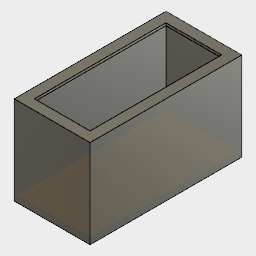
Doorbell_Casing_04 (Autodesk Fusion 360 design; units mm, degrees)
Autodesk Fusion 360 part; units mm, degrees
box "BoxPrimitive1" add length 60 width 30 height 35 placed x (0, 0, 1) y (1, 0, 0) z (0, 1, 0) at (0, 0, 0)
sketch "Sketch2" plane through (0, 35, 0) normal (0, 1, 0) x (-1, 0, 0)
  line L0 (0, 60) -> (-30, 60)
  line L1 (-30, 60) -> (-30, 0)
  line L2 (-30, 0) -> (0, 0)
  line L3 (0, 0) -> (0, 60)
  line L4 (-1, 0.9321) -> (-29, 0.9321)
  line L5 (-29, 0.9321) -> (-29, 58.9321)
  line L6 (-29, 58.9321) -> (-1, 58.9321)
  line L7 (-1, 58.9321) -> (-1, 0.9321)
  line L8 (-1, 0.9321) -> (-29, 58.9321) construction
  line L9 (-29, 0.9321) -> (-1, 58.9321) construction
  line L10 (-1, 58.9321) -> (-29, 58.9321)
  line L11 (-29, 58.9321) -> (-29, 0.9321)
  line L12 (-29, 0.9321) -> (-1, 0.9321)
  line L13 (-1, 0.9321) -> (-1, 58.9321)
  line L14 (30, 60) -> (0, 60)
  line L15 (0, 60) -> (0, 0)
  line L16 (0, 0) -> (30, 0)
  line L17 (30, 0) -> (30, 60)
  circle A0 centre (-15, 29.9346) radius 5
  line L18 (-1, 58.9321) -> (-29, 58.9321)
  line L19 (-29, 58.9321) -> (-29, 0.9321)
  line L20 (-29, 0.9321) -> (-1, 0.9321)
  line L21 (-1, 0.9321) -> (-1, 58.9321)
  circle A1 centre (15, 30) radius 4.5
  line L22 (30, 60) -> (0, 60)
  line L23 (0, 60) -> (0, 0)
  line L24 (0, 0) -> (30, 0)
  line L25 (30, 0) -> (30, 60)
  circle A2 centre (15, 40.0509) radius 2.5
  circle A3 centre (15, 30) radius 4.5
  line L26 (30, 60) -> (0, 60)
  line L27 (0, 60) -> (0, 0)
  line L28 (0, 0) -> (30, 0)
  line L29 (30, 0) -> (30, 60)
  circle A4 centre (14.9584, 19.9588) radius 2.5
  circle A5 centre (15, 40.0509) radius 2.5
  circle A6 centre (15, 30) radius 4.5
  line L30 (30, 60) -> (0, 60)
  line L31 (0, 60) -> (0, 0)
  line L32 (0, 0) -> (30, 0)
  line L33 (30, 0) -> (30, 60)
  circle A7 centre (14.893, 44.9593) radius 0.75
  circle A8 centre (14.9584, 19.9588) radius 2.5
  circle A9 centre (15, 40.0509) radius 2.5
  circle A10 centre (15, 30) radius 4.5
  line L34 (30, 60) -> (0, 60)
  line L35 (0, 60) -> (0, 0)
  line L36 (0, 0) -> (30, 0)
  line L37 (30, 0) -> (30, 60)
  line L38 (-29, 0.9321) -> (-29, 58.9321)
  line L39 (-29, 58.9321) -> (-1, 58.9321)
  line L40 (-1, 58.9321) -> (-1, 0.9321)
  line L41 (-1, 0.9321) -> (-29, 0.9321)
  line L42 (0, 60) -> (-30, 60)
  line L43 (-30, 60) -> (-30, 0)
  line L44 (-30, 0) -> (0, 0)
  line L45 (0, 0) -> (0, 60)
  line L46 (-29, 4) -> (-29, 58.9321)
  line L47 (-29, 58.9321) -> (-1, 58.9321)
  line L48 (-1, 58.9321) -> (-1, 4)
  line L49 (-1, 4) -> (-29, 4)
  line L50 (0, 60) -> (-30, 60)
  line L51 (-30, 60) -> (-30, 0)
  line L52 (-30, 0) -> (0, 0)
  line L53 (0, 0) -> (0, 60)
  line L54 (-29, 4) -> (-29, 56)
  line L55 (-29, 56) -> (-1, 56)
  line L56 (-1, 56) -> (-1, 4)
  line L57 (-1, 4) -> (-29, 4)
  line L58 (0, 60) -> (-30, 60)
  line L59 (-30, 60) -> (-30, 0)
  line L60 (-30, 0) -> (0, 0)
  line L61 (0, 0) -> (0, 60)
  line L62 (-29, 4) -> (-29, 56)
  line L63 (-29, 56) -> (-4, 56)
  line L64 (-4, 56) -> (-4, 4)
  line L65 (-4, 4) -> (-29, 4)
  line L66 (0, 60) -> (-30, 60)
  line L67 (-30, 60) -> (-30, 0)
  line L68 (-30, 0) -> (0, 0)
  line L69 (0, 0) -> (0, 60)
  dimension "d16" = 2
  dimension "d17" = 6.8
  dimension "d18" = 90
  constraint perpendicular L4 L5
  constraint parallel L4 L6
  constraint parallel L5 L7
  constraint horizontal L4
  constraint coincident L8
  constraint coincident L9
extrude "Extrude1" cut sketch "Sketch2" against normal blind 33 contours L4 L5 L7 L11 L12 L13 L19 L20 L21 L38 L40 L41 L49 L57 L65 | L7 L13 L21 L40 L48 L49 L55 L56 L57 L64 | L5 L11 L19 L38 L46 L49 L54 L55 L57 L62 L63 L64 L65 | L5 L6 L7 L10 L11 L13 L18 L19 L21 L38 L39 L40 L46 L47 L48 L55 L63 | A0
sketch "Sketch3" plane through (0, 2, 0) normal (0, 1, 0) x (-1, 0, 0)
  line L0 (-1, 58.9321) -> (-29, 58.9321)
  line L1 (-29, 58.9321) -> (-29, 0.9321)
  line L2 (-29, 0.9321) -> (-1, 0.9321)
  line L3 (-1, 0.9321) -> (-1, 58.9321)
  circle A0 centre (-15, 29.9346) radius 5
  dimension "d10" = 10
  measures "d10" diameter of A0
extrude "Extrude2" add sketch "Sketch3" along normal blind 6 contours A0
sketch "Sketch4" plane through (0, 0, 0) normal (0, -1, 0) x (1, 0, 0)
  line L0 (30, 60) -> (0, 60)
  line L1 (0, 60) -> (0, 0)
  line L2 (0, 0) -> (30, 0)
  line L3 (30, 0) -> (30, 60)
  circle A0 centre (15, 30) radius 4.5
  dimension "d13" = 9
  measures "d13" diameter of A0
extrude "Extrude3" cut sketch "Sketch4" against normal blind 5 contours A0
sketch "Sketch5" plane through (0, 2, 0) normal (0, 1, 0) x (-1, 0, 0)
  circle A0 centre (-15, 29.9346) radius 5
  line L0 (-1, 58.9321) -> (-29, 58.9321)
  line L1 (-29, 58.9321) -> (-29, 0.9321)
  line L2 (-29, 0.9321) -> (-1, 0.9321)
  line L3 (-1, 0.9321) -> (-1, 58.9321)
hole "Hole1" at (15, 8, 29.9346) direction (0, -1, 0) diameter 6.8 depth 2 tip angle 90
sketch "Sketch6" plane through (0, 0, 0) normal (0, -1, 0) x (1, 0, 0)
  circle A0 centre (15, 30) radius 4.5
  line L0 (30, 60) -> (0, 60)
  line L1 (0, 60) -> (0, 0)
  line L2 (0, 0) -> (30, 0)
  line L3 (30, 0) -> (30, 60)
  circle A1 centre (15, 40.0509) radius 2.5
  dimension "d19" = 5
  measures "d19" diameter of A1
extrude "Extrude4" cut sketch "Sketch6" against normal blind 2 contours A1
sketch "Sketch7" plane through (0, 0, 0) normal (0, -1, 0) x (1, 0, 0)
  circle A0 centre (15, 40.0509) radius 2.5
  circle A1 centre (15, 30) radius 4.5
  line L0 (30, 60) -> (0, 60)
  line L1 (0, 60) -> (0, 0)
  line L2 (0, 0) -> (30, 0)
  line L3 (30, 0) -> (30, 60)
  circle A2 centre (14.9584, 19.9588) radius 2.5
  dimension "d22" = 5
  measures "d22" diameter of A2
extrude "Extrude5" cut sketch "Sketch7" against normal blind 2 contours A2
sketch "Sketch8" plane through (0, 0, 0) normal (0, -1, 0) x (1, 0, 0)
  circle A0 centre (14.9584, 19.9588) radius 2.5
  circle A1 centre (15, 40.0509) radius 2.5
  circle A2 centre (15, 30) radius 4.5
  line L0 (30, 60) -> (0, 60)
  line L1 (0, 60) -> (0, 0)
  line L2 (0, 0) -> (30, 0)
  line L3 (30, 0) -> (30, 60)
  circle A3 centre (14.893, 44.9593) radius 0.75
  dimension "d25" = 1.5
  measures "d25" diameter of A3
extrude "Extrude6" cut sketch "Sketch8" against normal blind 2 contours A3
sketch "Sketch9" plane through (0, 0, 0) normal (0, -1, 0) x (1, 0, 0)
  circle A0 centre (14.893, 44.9593) radius 0.75
  circle A1 centre (14.9584, 19.9588) radius 2.5
  circle A2 centre (15, 40.0509) radius 2.5
  circle A3 centre (15, 30) radius 4.5
  line L0 (30, 60) -> (0, 60)
  line L1 (0, 60) -> (0, 0)
  line L2 (0, 0) -> (30, 0)
  line L3 (30, 0) -> (30, 60)
  circle A4 centre (15, 15.0503) radius 0.75
  dimension "d28" = 1.5
  measures "d28" diameter of A4
extrude "Extrude7" cut sketch "Sketch9" against normal blind 2 contours A4
sketch "Sketch10" plane through (0, 35, 0) normal (0, 1, 0) x (-1, 0, 0)
  line L0 (-29, 0.9321) -> (-29, 58.9321)
  line L1 (-29, 58.9321) -> (-1, 58.9321)
  line L2 (-1, 58.9321) -> (-1, 0.9321)
  line L3 (-1, 0.9321) -> (-29, 0.9321)
  line L4 (0, 60) -> (-30, 60)
  line L5 (-30, 60) -> (-30, 0)
  line L6 (-30, 0) -> (0, 0)
  line L7 (0, 0) -> (0, 60)
  line L8 (0, 0) -> (-30, 0)
  line L9 (-30, 0) -> (-30, 4)
  line L10 (-30, 4) -> (0, 4)
  line L11 (0, 4) -> (0, 0)
  dimension "d31" = 4
  constraint horizontal L8
  constraint vertical L9
  constraint horizontal L10
  constraint vertical L11
  constraint coincident L6.end L7.start
extrude "Extrude8" add sketch "Sketch10" against normal blind 1 contours L0 L2 L3 L10
sketch "Sketch11" plane through (0, 35, 0) normal (0, 1, 0) x (-1, 0, 0)
  line L0 (-29, 4) -> (-29, 58.9321)
  line L1 (-29, 58.9321) -> (-1, 58.9321)
  line L2 (-1, 58.9321) -> (-1, 4)
  line L3 (-1, 4) -> (-29, 4)
  line L4 (0, 60) -> (-30, 60)
  line L5 (-30, 60) -> (-30, 0)
  line L6 (-30, 0) -> (0, 0)
  line L7 (0, 0) -> (0, 60)
  line L8 (0, 60) -> (-30, 60)
  line L9 (-30, 60) -> (-30, 56)
  line L10 (-30, 56) -> (0, 56)
  line L11 (0, 56) -> (0, 60)
  dimension "d34" = 4
  dimension "d35" = 30
  constraint horizontal L8
  constraint vertical L9
  constraint horizontal L10
  constraint vertical L11
  constraint coincident L6.end L7.start
  measures "d34" distance of L6.end
extrude "Extrude9" add sketch "Sketch11" against normal blind 1 contours L0 L1 L2 L10
sketch "Sketch12" plane through (0, 35, 0) normal (0, 1, 0) x (-1, 0, 0)
  line L0 (-29, 4) -> (-29, 56)
  line L1 (-29, 56) -> (-1, 56)
  line L2 (-1, 56) -> (-1, 4)
  line L3 (-1, 4) -> (-29, 4)
  line L4 (0, 60) -> (-30, 60)
  line L5 (-30, 60) -> (-30, 0)
  line L6 (-30, 0) -> (0, 0)
  line L7 (0, 0) -> (0, 60)
  line L8 (0, 60) -> (-4, 60)
  line L9 (-4, 60) -> (-4, 0)
  line L10 (-4, 0) -> (0, 0)
  line L11 (0, 0) -> (0, 60)
  dimension "d38" = 4
  dimension "d39" = 60
  constraint horizontal L8
  constraint vertical L9
  constraint horizontal L10
  constraint vertical L11
  constraint coincident L6.end L7.start
extrude "Extrude10" add sketch "Sketch12" against normal blind 1 contours L1 L2 L3 L9
sketch "Sketch13" plane through (0, 35, 0) normal (0, 1, 0) x (-1, 0, 0)
  line L0 (-29, 4) -> (-29, 56)
  line L1 (-29, 56) -> (-4, 56)
  line L2 (-4, 56) -> (-4, 4)
  line L3 (-4, 4) -> (-29, 4)
  line L4 (0, 60) -> (-30, 60)
  line L5 (-30, 60) -> (-30, 0)
  line L6 (-30, 0) -> (0, 0)
  line L7 (0, 0) -> (0, 60)
  line L8 (-30, 0) -> (-26, 0)
  line L9 (-26, 0) -> (-26, 60)
  line L10 (-26, 60) -> (-30, 60)
  line L11 (-30, 60) -> (-30, 0)
  dimension "d42" = 4
  dimension "d43" = 60
  constraint horizontal L8
  constraint vertical L9
  constraint horizontal L10
  constraint vertical L11
  constraint coincident L6.end L7.start
extrude "Extrude11" add sketch "Sketch13" against normal blind 1 contours L0 L1 L3 L9
